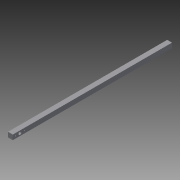
# Autodesk Inventor part: utilityarm1x1
Saved by Autodesk Inventor 2014 (Build 180170000, 170)
## iProperties
Created: 2014-01-16
Part Number: utilityarm1x1
Material: Generic
Document SubType Name: Modeling
Designer: pc
Density: 1 g/cm^3
Appearance: Default
Author: pc
Autodesk Inventor part; units mm, degrees
ref_plane "YZ Plane" through (0, 0, 0) normal (1, 0, 0) x (0, 1, 0)
ref_plane "XZ Plane" through (0, 0, 0) normal (0, 1, 0) x (-1, 0, 0)
ref_plane "XY Plane" through (0, 0, 0) normal (0, 0, 1) x (1, 0, 0)
sketch "Sketch1" plane through (0, 0, 0) normal (0, 0, 1) x (1, 0, 0)
  line L0 (0, 0) -> (25.4, 0)
  line L1 (25.4, 0) -> (25.4, 25.4)
  line L2 (25.4, 25.4) -> (0, 25.4)
  line L3 (0, 25.4) -> (0, 0)
  dimension "d0" = 25.4
  dimension "d1" = 25.4
  constraints: 8 end point, 2 parallel, 1 horizontal, 1 perpendicular
  measures "d0" distance of L2.end L1.end
  measures "d1" distance of L1.end L0.end
extrude "Extrusion1" add sketch "Sketch1" along normal blind 838.2
sketch "Sketch2" plane through (25.4, 0, 0) normal (1, 0, 0) x (0, 0, -1)
  line L0 (-838.2, 0) -> (-838.2, 25.4) projected
  circle A0 centre (-800.1, 12.7) radius 7.9375
  circle A1 centre (-823.9125, 12.7) radius 2.3813
  circle A2 centre (-776.2875, 12.7) radius 2.3812
  dimension "d4" = 15.875
  dimension "d5" = 38.1
  dimension "d8" = 4.7625
  dimension "d9" = 4.7625
  dimension "d10" = 23.8125
  dimension "d11" = 23.8125
  constraints: 3 centre point
  measures "d4" diameter of A0
  measures "d5" distance from line of L0 A0.centre
  measures "d8" diameter of A1
  measures "d9" diameter of A2
  measures "d10" distance of A0.centre A1.centre
  measures "d11" distance of A2.centre A0.centre
extrude "Extrusion3" cut sketch "Sketch2" against normal blind 25.4
equation "\"d11\" = d10"
body "Solid1"
